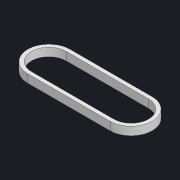
# Autodesk Inventor part: 70 Tooth Belt Around 36 Tooth Pulleys
Saved by Autodesk Inventor 2022 (Build 260153000, 153)
## iProperties
Created: 2022-09-18
Part Number: 70 Tooth Belt Around 36 Tooth Pulleys
Material: Generic
Document SubType Name: Modeling
Designer: robpl
Density: 1 g/cm^3
Appearance: Default
Author: robpl
Autodesk Inventor part; units mm, degrees
ref_plane "YZ Plane" through (0, 0, 0) normal (1, 0, 0) x (0, 1, 0)
ref_plane "XZ Plane" through (0, 0, 0) normal (0, 1, 0) x (-1, 0, 0)
ref_plane "XY Plane" through (0, 0, 0) normal (0, 0, 1) x (1, 0, 0)
sketch "Sketch1" plane through (0, 0, 0) normal (0, 1, 0) x (-1, 0, 0)
  line L0 (0, 0) -> (90, 0) construction
  line L1 (0, -19.099) -> (90, -19.099)
  line L2 (90, 19.099) -> (0, 19.099)
  arc A0 (0, 19.099) -> (0, -19.099) centre (0, 0) ccw
  arc A1 (90, -19.099) -> (90, 19.099) centre (90, 0) ccw
  line L3 (90, 23.099) -> (0, 23.099)
  arc A2 (0, 23.099) -> (0, -23.099) centre (0, 0) ccw
  line L4 (0, -23.099) -> (90, -23.099)
  arc A3 (90, -23.099) -> (90, 23.099) centre (90, 0) ccw
  point P0 (45, 0)
  dimension "d0" = 90
  dimension "d1" = 38.198
  dimension "d2" = 4
  constraints: 12 end point, 8 point on circle, 4 centre point, 4 tangent, 2 parallel, 1 horizontal, 1 midpoint, 3 other
  measures "d0" distance of L0.start L0.end
  measures "d1" diameter of A1
  measures "d2" radial gap between concentric circles of A1 A3
extrude "Extrusion1" add sketch "Sketch1" along normal blind 9
body "Solid1"
